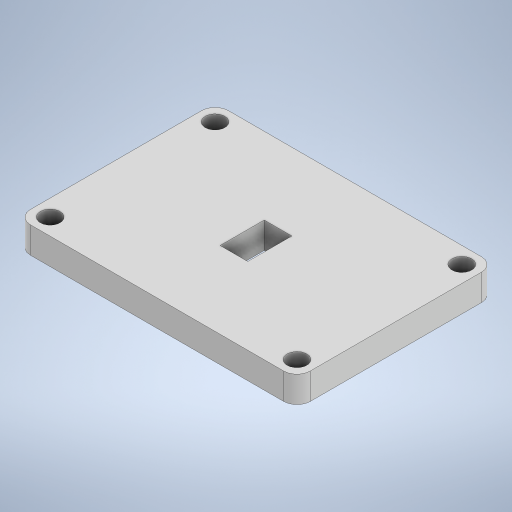
# Autodesk Inventor part: DAWN_motor_house_mold_lid
Saved by Autodesk Inventor 2024.3 (Build 283343000, 343)
## iProperties
Created: 2024-10-22
Part Number: DAWN_motor_house_mold_lid
Material: Generic
Document SubType Name: Modeling
Designer: magn1
Density: 1 g/cm^3
Appearance: Default
Author: magn1
Autodesk Inventor part; units mm, degrees
ref_plane "YZ Plane" through (0, 0, 0) normal (1, 0, 0) x (0, 1, 0)
ref_plane "XZ Plane" through (0, 0, 0) normal (0, 1, 0) x (-1, 0, 0)
ref_plane "XY Plane" through (0, 0, 0) normal (0, 0, 1) x (1, 0, 0)
sketch "Sketch1" plane through (0, 0, 0) normal (0, 1, 0) x (-1, 0, 0)
  line L0 (-18.714, 12.5) -> (18.714, 12.5) construction
  line L1 (18.714, 12.5) -> (18.714, -12.5) construction
  line L2 (18.714, -12.5) -> (-18.714, -12.5) construction
  line L3 (-18.714, -12.5) -> (-18.714, 12.5) construction
  line L4 (-18.714, 12.5) -> (18.714, -12.5) construction
  line L5 (18.714, 12.5) -> (-18.714, -12.5) construction
  circle A0 centre (18.714, -12.5) radius 1.5
  circle A1 centre (18.714, 12.5) radius 1.5
  circle A2 centre (-18.714, -12.5) radius 1.5
  circle A3 centre (-18.714, 12.5) radius 1.5
  line L6 (21.214, 15) -> (-21.214, 15)
  line L7 (-21.214, 15) -> (-21.214, -15)
  line L8 (-21.214, -15) -> (21.214, -15)
  line L9 (21.214, -15) -> (21.214, 15)
  line L10 (21.214, 15) -> (-21.214, -15) construction
  line L11 (-21.214, 15) -> (21.214, -15) construction
  line L12 (0.6, 1.85) -> (-0.6, 1.85) construction
  line L13 (-0.6, 1.85) -> (-0.6, -1.85) construction
  line L14 (-0.6, -1.85) -> (0.6, -1.85) construction
  line L15 (0.6, -1.85) -> (0.6, 1.85) construction
  line L16 (0.6, 1.85) -> (-0.6, -1.85) construction
  line L17 (-0.6, 1.85) -> (0.6, -1.85) construction
  line L18 (-2.1, 3.35) -> (2.1, 3.35)
  line L19 (2.1, 3.35) -> (2.1, -3.35)
  line L20 (2.1, -3.35) -> (-2.1, -3.35)
  line L21 (-2.1, -3.35) -> (-2.1, 3.35)
  line L22 (-2.1, 3.35) -> (2.1, -3.35) construction
  line L23 (2.1, 3.35) -> (-2.1, -3.35) construction
  point P0 (0, 0)
  dimension "d0" = 37.428
  dimension "d1" = 25
  dimension "d2" = 3
  dimension "d3" = 3
  dimension "d4" = 3
  dimension "d5" = 3
  dimension "d6" = 42.428
  dimension "d7" = 30
  dimension "d8" = 1.2
  dimension "d9" = 3.7
  dimension "d10" = 4.2
  dimension "d11" = 6.7
  constraints: 48 end point, 8 midpoint, 8 parallel, 4 centre point, 4 coincident, 4 horizontal, 4 perpendicular
  measures "d0" distance of L1.end L2.end
  measures "d1" distance of L0.end L1.end
  measures "d2" diameter of A0
  measures "d3" diameter of A1
  measures "d4" diameter of A2
  measures "d5" diameter of A3
  measures "d6" distance of L8.end L7.end
  measures "d7" distance of L7.end L6.end
  measures "d8" distance of L14.end L13.end
  measures "d9" distance of L13.end L12.end
  measures "d10" distance of L19.end L20.end
  measures "d11" distance of L18.end L19.end
extrude "Extrusion1" add sketch "Sketch1" along normal blind 4
fillet "Fillet1" radius 2 4 edges at (-21.214, 2, 15) (21.214, 2, 15) (21.214, 2, -15) (-21.214, 2, -15)
body "Solid1"
